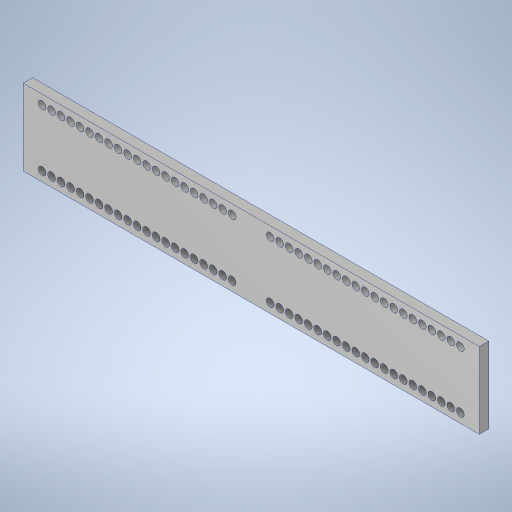
# Autodesk Inventor part: Gp1-001
Saved by Autodesk Inventor 2023.4 (Build 274418000, 418)
## iProperties
Created: 2025-01-05
Part Number: Gp1-001
Material: Aluminum 6061
Document SubType Name: Modeling
Designer: mavericks
Density: 2.7 g/cm^3
Appearance: Aluminum - Flat
Author: mavericks
Autodesk Inventor part; units mm, degrees
ref_plane "YZ Plane" through (0, 0, 0) normal (1, 0, 0) x (0, 1, 0)
ref_plane "XZ Plane" through (0, 0, 0) normal (0, 1, 0) x (-1, 0, 0)
ref_plane "XY Plane" through (0, 0, 0) normal (0, 0, 1) x (1, 0, 0)
sketch "Sketch1" plane through (0, 0, 0) normal (0, 0, 1) x (1, 0, 0)
  line L0 (-152.4, 25.4) -> (152.4, 25.4)
  line L1 (152.4, 25.4) -> (152.4, -25.4)
  line L2 (152.4, -25.4) -> (-152.4, -25.4)
  line L3 (-152.4, -25.4) -> (-152.4, 25.4)
  line L4 (-152.4, 25.4) -> (152.4, -25.4) construction
  line L5 (152.4, 25.4) -> (-152.4, -25.4) construction
  point P0 (0, 0)
  dimension "d0" = 304.8
  dimension "d1" = 50.8
  constraints: 12 end point, 2 midpoint, 2 parallel, 1 horizontal, 1 perpendicular
  measures "d0" distance of L1.end L2.end
  measures "d1" distance of L0.end L1.end
extrude "Extrusion1" add sketch "Sketch1" along normal blind 6.35
sketch "Sketch2" plane through (0, 0, 6.35) normal (0, 0, 1) x (1, 0, 0)
  line L0 (-152.4, 25.4) -> (-152.4, -25.4) construction
  line L1 (152.4, 25.4) -> (-152.4, 25.4) construction
  line L2 (-43.7106, 0) -> (44.45, 0) construction
  line L3 (-152.4, -25.4) -> (152.4, -25.4) construction
  line L4 (0, 17.6576) -> (0, -13.3598) construction
  point P0 (0, 0)
  point P1 (-139.7, 19.05)
  point P2 (-133.35, 19.05)
  point P3 (-127, 19.05)
  point P4 (-120.65, 19.05)
  point P5 (-114.3, 19.05)
  point P6 (-107.95, 19.05)
  point P7 (-101.6, 19.05)
  point P8 (-95.25, 19.05)
  point P9 (-88.9, 19.05)
  point P10 (-82.55, 19.05)
  point P11 (-76.2, 19.05)
  point P12 (-69.85, 19.05)
  point P13 (-63.5, 19.05)
  point P14 (-57.15, 19.05)
  point P15 (-50.8, 19.05)
  point P16 (-44.45, 19.05)
  point P17 (-38.1, 19.05)
  point P18 (-31.75, 19.05)
  point P19 (-25.4, 19.05)
  point P20 (-19.05, 19.05)
  point P21 (-12.7, 19.05)
  point P22 (-139.7, -19.05)
  point P23 (-133.35, -19.05)
  point P24 (-127, -19.05)
  point P25 (-120.65, -19.05)
  point P26 (-114.3, -19.05)
  point P27 (-107.95, -19.05)
  point P28 (-101.6, -19.05)
  point P29 (-95.25, -19.05)
  point P30 (-88.9, -19.05)
  point P31 (-82.55, -19.05)
  point P32 (-76.2, -19.05)
  point P33 (-69.85, -19.05)
  point P34 (-63.5, -19.05)
  point P35 (-57.15, -19.05)
  point P36 (-50.8, -19.05)
  point P37 (-44.45, -19.05)
  point P38 (-38.1, -19.05)
  point P39 (-31.75, -19.05)
  point P40 (-25.4, -19.05)
  point P41 (-19.05, -19.05)
  point P42 (-12.7, -19.05)
  point P43 (139.7, 19.05)
  point P44 (133.35, 19.05)
  point P45 (127, 19.05)
  point P46 (120.65, 19.05)
  point P47 (114.3, 19.05)
  point P48 (107.95, 19.05)
  point P49 (101.6, 19.05)
  point P50 (95.25, 19.05)
  point P51 (88.9, 19.05)
  point P52 (82.55, 19.05)
  point P53 (76.2, 19.05)
  point P54 (69.85, 19.05)
  point P55 (63.5, 19.05)
  point P56 (57.15, 19.05)
  point P57 (50.8, 19.05)
  point P58 (44.45, 19.05)
  point P59 (38.1, 19.05)
  point P60 (31.75, 19.05)
  point P61 (25.4, 19.05)
  point P62 (19.05, 19.05)
  point P63 (12.7, 19.05)
  point P64 (43.7106, 0)
  point P65 (12.7, -19.05)
  point P66 (19.05, -19.05)
  point P67 (25.4, -19.05)
  point P68 (31.75, -19.05)
  point P69 (38.1, -19.05)
  point P70 (44.45, -19.05)
  point P71 (50.8, -19.05)
  point P72 (57.15, -19.05)
  point P73 (63.5, -19.05)
  point P74 (69.85, -19.05)
  point P75 (76.2, -19.05)
  point P76 (82.55, -19.05)
  point P77 (88.9, -19.05)
  point P78 (95.25, -19.05)
  point P79 (101.6, -19.05)
  point P80 (107.95, -19.05)
  point P81 (114.3, -19.05)
  point P82 (120.65, -19.05)
  point P83 (127, -19.05)
  point P84 (133.35, -19.05)
  point P85 (139.7, -19.05)
  point P86 (0, 2.1489)
  dimension "d4" = 12.7
  dimension "d5" = 6.35
  dimension "d8" = 6.35
  dimension "d13" = 6.35
  constraints: 64 symmetric about line, 4 end point, 2 horizontal, 1 midpoint, 1 vertical, 1 vertical alignment, 20 other
  measures "d4" distance from line of point (-139.7, 19.05) L0
  measures "d5" distance from line of point (-139.7, 19.05) L1
  measures "d8" distance of point (-139.7, 19.05) point (-133.35, 19.05)
  measures "d13" distance from line of L3 point (-139.7, -19.05)
hole "Hole1" at (-139.7, 19.05, 6.35) at (-133.35, 19.05, 6.35) at (-127, 19.05, 6.35) at (-120.65, 19.05, 6.35) at (-114.3, 19.05, 6.35) at (-107.95, 19.05, 6.35) at (-101.6, 19.05, 6.35) at (-95.25, 19.05, 6.35) at (-88.9, 19.05, 6.35) at (-82.55, 19.05, 6.35) at (-76.2, 19.05, 6.35) at (-69.85, 19.05, 6.35) at (-63.5, 19.05, 6.35) at (-57.15, 19.05, 6.35) at (-50.8, 19.05, 6.35) at (-44.45, 19.05, 6.35) at (-38.1, 19.05, 6.35) at (-31.75, 19.05, 6.35) at (-25.4, 19.05, 6.35) at (-19.05, 19.05, 6.35) at (-12.7, 19.05, 6.35) at (-12.7, -19.05, 6.35) at (-19.05, -19.05, 6.35) at (-25.4, -19.05, 6.35) at (-31.75, -19.05, 6.35) at (-38.1, -19.05, 6.35) at (-44.45, -19.05, 6.35) at (-50.8, -19.05, 6.35) at (-57.15, -19.05, 6.35) at (-63.5, -19.05, 6.35) at (-69.85, -19.05, 6.35) at (-76.2, -19.05, 6.35) at (-82.55, -19.05, 6.35) at (-88.9, -19.05, 6.35) at (-95.25, -19.05, 6.35) at (-101.6, -19.05, 6.35) at (-107.95, -19.05, 6.35) at (-114.3, -19.05, 6.35) at (-120.65, -19.05, 6.35) at (-127, -19.05, 6.35) at (-133.35, -19.05, 6.35) at (-139.7, -19.05, 6.35) at (12.7, 19.05, 6.35) at (12.7, -19.05, 6.35) at (19.05, -19.05, 6.35) at (25.4, -19.05, 6.35) at (31.75, -19.05, 6.35) at (38.1, -19.05, 6.35) at (44.45, -19.05, 6.35) at (50.8, -19.05, 6.35) direction (0, 0, -1) diameter 5.1054 end through all and at (57.15, -19.05, 6.35) (63.5, -19.05, 6.35) (69.85, -19.05, 6.35) (76.2, -19.05, 6.35) (82.55, -19.05, 6.35) (88.9, -19.05, 6.35) (95.25, -19.05, 6.35) (101.6, -19.05, 6.35) (107.95, -19.05, 6.35) (114.3, -19.05, 6.35) (120.65, -19.05, 6.35) (127, -19.05, 6.35) (133.35, -19.05, 6.35) (139.7, -19.05, 6.35) (139.7, 19.05, 6.35) (133.35, 19.05, 6.35) (127, 19.05, 6.35) (120.65, 19.05, 6.35) (114.3, 19.05, 6.35) (107.95, 19.05, 6.35) (101.6, 19.05, 6.35) (95.25, 19.05, 6.35) (88.9, 19.05, 6.35) (82.55, 19.05, 6.35) (76.2, 19.05, 6.35) (69.85, 19.05, 6.35) (63.5, 19.05, 6.35) (57.15, 19.05, 6.35) (50.8, 19.05, 6.35) (44.45, 19.05, 6.35) (38.1, 19.05, 6.35) (31.75, 19.05, 6.35) (25.4, 19.05, 6.35) (19.05, 19.05, 6.35) clearance for "Flat Head Machine Screw (82)" size "#10" standard "Ansi Unified Screw Threads"
body "Solid1"
